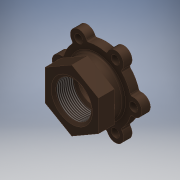
# Autodesk Inventor part: Body Cap
Saved by Autodesk Inventor 2018 (Build 220112000, 112)
## iProperties
Created: 2016-08-30
Part Number: Body Cap
Material: Bronze, Soft Tin
Document SubType Name: Modeling
Designer: zxiang3
Density: 8.874 g/cm^3
Appearance: Bronze - Satin
Author: zxiang3
Autodesk Inventor part; units mm, degrees
ref_plane "YZ Plane" through (0, 0, 0) normal (1, 0, 0) x (0, 1, 0)
ref_plane "XZ Plane" through (0, 0, 0) normal (0, 1, 0) x (-1, 0, 0)
ref_plane "XY Plane" through (0, 0, 0) normal (0, 0, 1) x (1, 0, 0)
sketch "Sketch1" plane through (0, 0, 0) normal (0, 0, 1) x (1, 0, 0)
  line L0 (0, -7.8) -> (0, 46.8) projected
  line L1 (19, 21) -> (19, 2)
  line L2 (22, 0) -> (28.5, 0)
  line L3 (19, 2) -> (22, 0)
  line L4 (-7.4, 0) -> (44.4, 0) projected
  line L5 (19, 21) -> (16, 23)
  line L6 (16, 23) -> (16, 26)
  line L7 (16, 26) -> (20, 26)
  line L8 (20, 26) -> (20, 29)
  line L9 (20, 29) -> (25.5, 29)
  line L10 (25.5, 29) -> (25.5, 39)
  line L11 (25.5, 39) -> (28.5, 39)
  line L12 (28.5, 39) -> (28.5, 33)
  line L13 (28.5, 33) -> (33.5, 33)
  line L14 (33.5, 33) -> (33.5, 36)
  line L15 (33.5, 36) -> (37, 36)
  line L16 (37, 36) -> (37, 27)
  line L17 (37, 27) -> (28.5, 27)
  line L18 (28.5, 27) -> (28.5, 0)
  point P0 (0, 0)
  dimension "d2" = 38
  dimension "d3" = 57
  dimension "d4" = 3
  dimension "d6" = 2
  dimension "d7" = 21
  dimension "d8" = 26
  dimension "d9" = 23
  dimension "d10" = 40
  dimension "d12" = 29
  dimension "d13" = 51
  dimension "d14" = 57
  dimension "d15" = 5
  dimension "d16" = 27
  dimension "d17" = 33
  dimension "d18" = 36
  dimension "d19" = 39
  dimension "d20" = 74
  dimension "d22" = 32
  constraints: 34 end point, 8 perpendicular, 4 horizontal, 4 vertical
  measures "d2" diameter of L1 L0
  measures "d3" diameter of L2.end L0
  measures "d4" horizontal distance of L2.start L1.end
  measures "d6" vertical distance of L1.end L2.start
  measures "d7" distance from line of L4 L1.start
  measures "d8" distance from line of L4 L6.end
  measures "d9" distance from line of L4 L5.end
  measures "d10" diameter of L8 L0
  measures "d12" distance between parallel lines of L4 L9
  measures "d13" diameter of L10 L0
  measures "d14" diameter of L11.end L0
  measures "d15" distance of L12.end L13.end
  measures "d16" distance between parallel lines of L4 L17
  measures "d17" distance between parallel lines of L4 L13
  measures "d18" distance between parallel lines of L4 L15
  measures "d19" distance between parallel lines of L4 L11
  measures "d20" diameter of L16 L0
  measures "d22" diameter of L6 L0
revolve "Revolution1" add sketch "Sketch1" angle 360 about axis through (0, -10, 0) along (0, 1, 0)
thread "Thread1" size "M39x2" class "6H" standard "ANSI Metric M Profile" full length
sketch "Sketch2" plane through (0, 0, 0) normal (0, -1, 0) x (1, 0, 0)
  line L0 (0, 32.909) -> (28.5, 16.4545)
  line L1 (28.5, 16.4545) -> (28.5, -16.4545)
  line L2 (28.5, -16.4545) -> (0, -32.909)
  line L3 (0, -32.909) -> (-28.5, -16.4545)
  line L4 (-28.5, -16.4545) -> (-28.5, 16.4545)
  line L5 (-28.5, 16.4545) -> (0, 32.909)
  circle A0 centre (0, 0) radius 28.5
  dimension "d24" = 57
  constraints: 12 end point, 2 coincident, 1 centre point, 1 tangent, 1 vertical, 13 other
  measures "d24" distance between parallel lines of L1 L4
extrude "Extrusion1" add sketch "Sketch2" against normal blind 17 contours L0 A0 L5 | L0 L1 A0 | A0 L4 L5 | L1 L2 A0 | A0 L3 L4 | L2 L3 A0
sketch "Sketch3" plane through (0, 36, 0) normal (0, 1, 0) x (1, 0, 0)
  line L0 (0, 0) -> (24.2959, 42.0818) construction
  line L1 (0, 0) -> (48.5919, 0) construction
  circle A0 centre (0, 0) radius 39 construction
  circle A1 centre (19.5, 33.775) radius 4.5
  circle A2 centre (19.5, 33.775) radius 9
  circle A3 centre (0, 0) radius 33.5 projected
  arc A4 (-32.8494, -6.5704) -> (-22.1148, -25.1632) centre (0, 0) ccw
  circle A5 centre (-19.5, 33.775) radius 9
  circle A6 centre (-19.5, 33.775) radius 4.5
  circle A7 centre (-39, 0) radius 9
  circle A8 centre (-39, 0) radius 4.5
  circle A9 centre (-19.5, -33.775) radius 9
  circle A10 centre (-19.5, -33.775) radius 4.5
  circle A11 centre (19.5, -33.775) radius 9
  circle A12 centre (19.5, -33.775) radius 4.5
  circle A13 centre (39, 0) radius 9
  circle A14 centre (39, 0) radius 4.5
  arc A15 (-21.7914, 29.9021) -> (-36.7917, 3.9209) centre (0, 0) ccw
  arc A16 (-32.8494, 6.5704) -> (-33.5, 0) centre (0, 0) ccw
  arc A17 (-10.7346, 31.7336) -> (-22.1148, 25.1632) centre (0, 0) ccw
  arc A18 (-22.1148, 25.1632) -> (-32.8494, 6.5704) centre (0, 0) ccw
  arc A19 (10.7346, 31.7336) -> (-10.7346, 31.7336) centre (0, 0) ccw
  arc A20 (22.1148, 25.1632) -> (10.7346, 31.7336) centre (0, 0) ccw
  arc A21 (32.8494, 6.5704) -> (22.1148, 25.1632) centre (0, 0) ccw
  arc A22 (32.8494, -6.5704) -> (32.8494, 6.5704) centre (0, 0) ccw
  arc A23 (22.1148, -25.1632) -> (32.8494, -6.5704) centre (0, 0) ccw
  arc A24 (10.7346, -31.7336) -> (22.1148, -25.1632) centre (0, 0) ccw
  arc A25 (-10.7346, -31.7336) -> (10.7346, -31.7336) centre (0, 0) ccw
  arc A26 (-22.1148, -25.1632) -> (-10.7346, -31.7336) centre (0, 0) ccw
  arc A27 (-33.5, 0) -> (-32.8494, -6.5704) centre (0, 0) ccw
  arc A28 (-15.0003, 33.823) -> (-21.7914, 29.9021) centre (0, 0) ccw
  arc A29 (21.7914, 29.9021) -> (15.0003, 33.823) centre (0, 0) ccw
  arc A30 (15.0003, 33.823) -> (-15.0003, 33.823) centre (0, 0) ccw
  arc A31 (36.7917, 3.9209) -> (21.7914, 29.9021) centre (0, 0) ccw
  arc A32 (36.7917, -3.9209) -> (36.7917, 3.9209) centre (0, 0) ccw
  arc A33 (15.0003, -33.823) -> (21.7914, -29.9021) centre (0, 0) ccw
  arc A34 (21.7914, -29.9021) -> (36.7917, -3.9209) centre (0, 0) ccw
  arc A35 (-15.0003, -33.823) -> (15.0003, -33.823) centre (0, 0) ccw
  arc A36 (-21.7914, -29.9021) -> (-15.0003, -33.823) centre (0, 0) ccw
  arc A37 (-36.7917, -3.9209) -> (-21.7914, -29.9021) centre (0, 0) ccw
  arc A38 (-36.7917, 3.9209) -> (-36.7917, -3.9209) centre (0, 0) ccw
  dimension "d30" = 78
  dimension "d29" = 60
  dimension "d31" = 9
  dimension "d32" = 18
  dimension "d33" = 67
  dimension "d37" = 360
  dimension "d40" = 74
  constraints: 74 point on circle, 37 centre point, 8 coincident, 4 end point, 2 point on line, 1 concentric, 1 equal length, 1 horizontal, 28 other
  measures "d29" angle of L1 L0
  measures "d31" diameter of A1
  measures "d32" diameter of A2
  measures "d33" diameter of A4
  measures "d40" diameter of A15
extrude "Extrusion2" add sketch "Sketch3" against normal blind 9 contours A1 A30 A2 A31 | A1 A31 A2 A3 A30 | A30 A6 A15 A5 | A5 A3 A15 A6 A30 | A31 A14 A34 A13 A3 | A13 A34 A14 A31 | A15 A8 A37 A7 | A7 A3 A37 A8 A15 | A11 A34 A12 A35 A3 | A11 A35 A12 A34 | A37 A10 A35 A9 | A9 A3 A35 A10 A37
extrude "Extrusion3" cut sketch "Sketch3" against normal blind 9 contours A29 A1 | A6 A28 | A32 A14 | A8 A38 | A33 A12 | A10 A36 picked at (18.2331, 31.2289) picked at (-17.9356, 31.3995) picked at (36.1616, 0.1759) picked at (-36.1512, 0) picked at (18.2331, -31.2289) picked at (-17.9356, -31.3995)
fillet "Fillet1" radius 2 13 edges at (36.0128, 31.5, -8.4898) (36.0128, 31.5, 8.4898) (25.3588, 31.5, 26.9431) (10.654, 31.5, 35.4329) (-10.654, 31.5, 35.4329) (-25.3588, 31.5, 26.9431) (25.3588, 31.5, -26.9431) (10.654, 31.5, -35.4329) (-10.654, 31.5, -35.4329) (-25.3588, 31.5, -26.9431) (-36.0128, 31.5, -8.4898) (-36.0128, 31.5, 8.4898) (-28.5, 27, 0)
body "Solid1"
